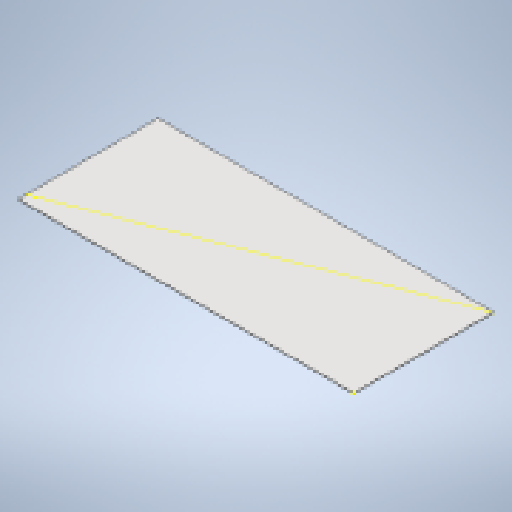
# Autodesk Inventor part: taringle
Saved by Autodesk Inventor 2025.2 (Build 292293000, 293)
## iProperties
Created: 2025-05-26
Part Number: taringle
Material: Generic
Document SubType Name: Sheet Metal
Designer: abdal
Density: 1 g/cm^3
Sheet Metal Rule: Default_mm
Appearance: Default
Author: abdal
Autodesk Inventor part; units mm, degrees
ref_plane "YZ Plane" through (0, 0, 0) normal (1, 0, 0) x (0, 1, 0)
ref_plane "XZ Plane" through (0, 0, 0) normal (0, 1, 0) x (-1, 0, 0)
ref_plane "XY Plane" through (0, 0, 0) normal (0, 0, 1) x (1, 0, 0)
sketch "Sketch1" plane through (0, 0, 0) normal (0, 1, 0) x (-1, 0, 0)
  line L0 (0, 0) -> (1020, 0)
  line L1 (0, -425.23) -> (0, 0)
  line L2 (1020, 0) -> (1020, -425.23)
  line L3 (1020, -425.23) -> (0, -425.23)
  dimension "d0" = 425.23
  dimension "d1" = 1020
  measures "d0" distance of L1.start L0.start
  measures "d1" distance of L0.start L0.end
extrude "Plate1" add sketch "Sketch1" along normal blind 2
sketch "Sketch2" plane through (0, 0, 0) normal (0, -1, 0) x (1, 0, 0)
  line L0 (0, -425.2298) -> (-1007.836, -30) projected
  line L1 (-996, -30) -> (-1014, -30) projected
  arc A0 (-1020, -24) -> (-1014, -30) centre (-1014, -24) ccw projected
  line L2 (0, -425.23) -> (-1020, -425.23) projected
  line L3 (0, 0) -> (0, -425.23) projected
  line L4 (-1020, 0) -> (0, 0) projected
  line L5 (-1020, -425.23) -> (-1020, 0) projected
extrude "Extrusion1" cut sketch "Sketch2" against normal through all contours L2 L5 A0 L1 L0
equation "\"d2\" = Thickness"
equation "\"BendRadius\" = Thickness"
equation "\"BendReliefWidth\" = Thickness"
equation "\"BendReliefDepth\" = 0.5 * Thickness"
equation "\"CornerReliefSize\" = 4 * Thickness"
equation "\"MinimumRemnant\" = 2 * Thickness"
equation "\"TransitionRadius\" = BendRadius"
equation "\"JacobiRadiusSize\" = BendRadius"
equation "\"GapSize\" = Thickness"
equation "\"Thickness\" = 2"
body "Solid1"
